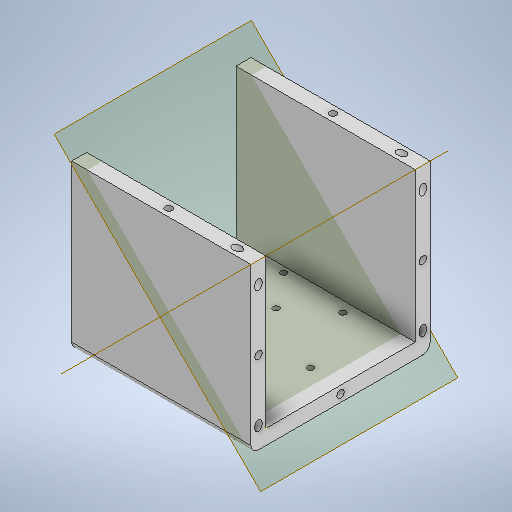
# Autodesk Inventor part: Fuselage_Body_Piece_Front
Saved by Autodesk Inventor 2025.1 (Build 291241020, 241B)
## iProperties
Created: 2025-02-15
Part Number: Fuselage_Body_Piece_Front
Material: Generic
Document SubType Name: Modeling
Designer: smyth
Density: 1 g/cm^3
Appearance: Default
Author: smyth
Autodesk Inventor part; units mm, degrees
ref_plane "YZ Plane" through (0, 0, 0) normal (1, 0, 0) x (0, 1, 0)
ref_plane "XZ Plane" through (0, 0, 0) normal (0, 1, 0) x (-1, 0, 0)
ref_plane "XY Plane" through (0, 0, 0) normal (0, 0, 1) x (1, 0, 0)
sketch "Sketch1" plane through (0, 0, 0) normal (0, 1, 0) x (-1, 0, 0)
  point P0 (0, 0)
sketch "Sketch2" plane through (0, 0, 0) normal (0, 1, 0) x (-1, 0, 0)
  line L0 (-76.2, 76.2) -> (76.2, 76.2)
  line L1 (76.2, 76.2) -> (76.2, -76.2)
  line L2 (76.2, -76.2) -> (-76.2, -76.2)
  line L3 (-76.2, -76.2) -> (-76.2, 76.2)
  line L4 (-76.2, 76.2) -> (76.2, -76.2) construction
  line L5 (76.2, 76.2) -> (-76.2, -76.2) construction
  point P0 (0, 0)
  dimension "d0" = 152.4
  dimension "d1" = 152.4
  constraints: 12 end point, 2 midpoint, 2 parallel, 1 horizontal, 1 perpendicular
  measures "d0" distance of L1.end L2.end
  measures "d1" distance of L0.end L1.end
extrude "Extrusion1" add sketch "Sketch2" along normal blind 12.7
sketch "Sketch3" plane through (0, 12.7, 0) normal (0, 1, 0) x (1, 0, 0)
  line L0 (76.2, 76.2) -> (-76.2, 76.2) projected
  line L1 (76.2, -76.2) -> (76.2, 76.2) projected
  line L2 (-76.2, 76.2) -> (76.2, 76.2)
  line L3 (76.2, 76.2) -> (76.2, 63.5)
  line L4 (76.2, 63.5) -> (-76.2, 63.5)
  line L5 (-76.2, 63.5) -> (-76.2, 76.2)
  line L6 (-76.2, -76.2) -> (76.2, -76.2)
  line L7 (76.2, -76.2) -> (76.2, -63.5)
  line L8 (76.2, -63.5) -> (-76.2, -63.5)
  line L9 (-76.2, -63.5) -> (-76.2, -76.2)
  point P0 (0, 0)
  point P1 (76.2, -76.2)
  dimension "d4" = 12.7
  dimension "d5" = 12.7
  dimension "d15" = 152.4
  constraints: 16 end point, 4 parallel, 2 horizontal, 2 perpendicular, 2 point on line
  measures "d4" distance between parallel lines of L4 L0
  measures "d5" distance between parallel lines of L8 L6
  measures "d15" distance of L6.start L6.end
extrude "Extrusion2" add sketch "Sketch3" along normal blind 127
fillet "Fillet1" radius 6.35 2 edges at (0, 0, 76.2) (0, 0, -76.2)
sketch "Sketch4" plane through (76.2, 12.7, -63.5) normal (1, 0, 0) x (0, 0, -1)
  circle A0 centre (-133.35, 57.15) radius 3.175
  circle A1 centre (6.35, 57.15) radius 3.175
  circle A2 centre (-63.5, -6.35) radius 3.175
  point P0 (-63.5, -12.7)
  constraints: 3 centre point
extrude "Extrusion3" cut sketch "Sketch4" against normal blind 12.7
sketch "Sketch5" plane through (-76.2, 12.7, 63.5) normal (-1, 0, 0) x (0, 0, 1)
  circle A0 centre (-133.35, 120.65) radius 3.175
  circle A1 centre (-133.35, 57.15) radius 3.175 projected
  circle A2 centre (-133.35, 57.15) radius 3.175
  circle A3 centre (-133.35, -6.35) radius 3.175
  circle A4 centre (-63.5, -6.35) radius 3.175 projected
  circle A5 centre (-63.5, -6.35) radius 3.175
  circle A6 centre (6.35, -6.35) radius 3.175
  circle A7 centre (6.35, 57.15) radius 3.175 projected
  circle A8 centre (6.35, 57.15) radius 3.175
  circle A9 centre (6.35, 120.65) radius 3.175
  line L0 (6.35, -12.7) -> (-133.35, -12.7) projected
  point P0 (-63.5, -12.7)
  point P1 (-133.35, 120.65)
  point P2 (-133.35, -6.35)
  point P3 (6.35, -6.35)
  point P4 (6.35, 120.65)
  dimension "d20" = 69.85
  constraints: 7 centre point, 7 coincident
  measures "d20" distance from line of L0 A8.centre
sketch "Sketch6" plane through (0, 139.7, 0) normal (0, 1, 0) x (1, 0, 0)
  line L0 (76.2, 69.85) -> (-76.2, 69.85) projected
  circle A0 centre (0, 69.85) radius 3
  line L1 (-76.2, -69.85) -> (76.2, -69.85) projected
  circle A1 centre (0, -69.85) radius 3
  point P0 (0, 0)
  dimension "d16" = 6
  dimension "d17" = 6
  constraints: 2 centre point, 2 midpoint
  measures "d16" diameter of A0
  measures "d17" diameter of A1
extrude "Extrusion5" cut sketch "Sketch6" against normal blind 4
extrude "Extrusion6" cut sketch "Sketch5" against normal blind 12.7 contours A1 | A4 | A7
ref_plane "Work Plane1" through (76.2, 139.7, 76.2) normal (0.7071, -0.7071, 0) x (0, 0, -1)
sketch "Sketch7" plane through (76.2, 139.7, 76.2) normal (0.7071, -0.7071, 0) x (0, 0, -1)
  line L0 (139.7, 0) -> (152.4, 0) projected
  line L1 (146.05, 0) -> (146.05, -12.7)
  circle A0 centre (146.05, -12.7) radius 3.175
  line L2 (0, 0) -> (12.7, 0) projected
  line L3 (6.35, 0) -> (6.35, -12.7)
  circle A1 centre (6.35, -12.7) radius 3.175
  point P0 (76.2, -152.6644)
  dimension "d24" = 12.7
  constraints: 4 end point, 2 centre point, 2 coincident, 2 midpoint, 2 vertical
  measures "d24" distance of L3.start L3.end
extrude "Extrusion7" cut sketch "Sketch7" along normal blind 31.75 and the other way blind 25.4
ref_plane "Work Plane2" through (76.2, 0, 76.2) normal (-0.7071, -0.7071, 0) x (0, 0, -1)
sketch "Sketch8" plane through (76.2, 0, 76.2) normal (-0.7071, -0.7071, 0) x (0, 0, -1)
  line L0 (6.35, 0) -> (146.05, 0) projected
  line L1 (146.05, 0) -> (146.05, -12.7)
  line L2 (146.05, 0) -> (146.05, -107.7631) projected
  line L3 (6.35, 0) -> (6.35, -12.7)
  line L4 (6.35, -107.7631) -> (6.35, 0) projected
  circle A0 centre (146.05, -12.7) radius 3.175
  circle A1 centre (6.35, -12.7) radius 3.175
  point P0 (76.2, -53.8815)
  dimension "d30" = 12.7
  dimension "d31" = 12.7
  constraints: 4 end point, 2 centre point, 2 coincident, 2 point on line
  measures "d30" distance of L0.end L1.end
  measures "d31" distance of L0.start L3.end
extrude "Extrusion8" cut sketch "Sketch8" along normal blind 25.4 and the other way blind 31.75
sketch "Sketch10" plane through (0, 12.7, 0) normal (0, 1, 0) x (1, 0, 0)
  line L0 (76.2, -63.5) -> (76.2, 63.5) projected
  line L1 (76.2, 0) -> (50.8, 0)
  circle A0 centre (50.8, 0) radius 2.6035
  line L2 (48.1965, 0) -> (-5.1435, 0)
  circle A1 centre (-7.747, 0) radius 2.6035
  line L3 (-5.1435, -17.8483) -> (-5.1435, 18.0947)
  line L4 (-5.1435, 0) -> (-5.1435, -49.2125)
  line L5 (23.8125, 0) -> (23.8125, -51.8414)
  line L6 (23.8125, 0) -> (23.8125, 51.8414)
  circle A2 centre (23.8125, -54.4449) radius 2.6035
  circle A3 centre (23.8125, 54.4449) radius 2.6035
  line L7 (30.1625, -51.8414) -> (15.875, -51.8414)
  line L8 (30.1625, 51.8414) -> (17.4625, 51.8414)
  point P0 (0, 0)
  dimension "d37" = 5.207
  dimension "d36" = 25.4
  dimension "d39" = 5.207
  dimension "d40" = 49.2125
  dimension "d41" = 51.8414
  dimension "d42" = 51.8414
  dimension "d43" = 5.207
  constraints: 16 end point, 4 horizontal, 3 centre point, 3 point on line, 3 tangent, 1 coincident, 1 horizontal alignment, 1 midpoint, 1 perpendicular, 1 vertical, 2 other
  measures "d36" distance of L1.start L1.end
  measures "d39" diameter of A1
  measures "d40" distance of L2.end L4.end
  measures "d41" distance of L5.start L5.end
  measures "d42" distance of L5.start L6.end
  measures "d43" diameter of A2
extrude "Extrusion9" cut sketch "Sketch10" against normal blind 3.9878
sketch "Sketch11" plane through (0, 12.7, 0) normal (0, 1, 0) x (1, 0, 0)
  circle A0 centre (-7.747, 0) radius 2.6035 projected
  line L0 (-10.3505, 29.2735) -> (-50.9905, 29.2735)
  line L1 (-63.5, -3.175) -> (-63.5, 3.175) projected
  line L2 (-50.8997, 16.5035) -> (-50.8997, 42.0435)
  circle A1 centre (-53.5032, 29.2735) radius 2.6035
  line L3 (-30.6705, 29.2735) -> (-30.6705, 2.6035)
  line L4 (-30.6705, 29.2735) -> (-30.6705, 55.9435)
  line L5 (-23.5267, 29.2578) -> (-40.9893, 29.2578)
  line L6 (-40.9893, 2.6035) -> (-17.4625, 2.6035)
  circle A2 centre (-30.6705, 0) radius 2.6035
  line L7 (-37.2049, 55.9435) -> (-23.5267, 55.9435)
  circle A3 centre (-30.6705, 58.547) radius 2.6035
  circle A4 centre (-7.747, 29.2578) radius 2.6035
  point P0 (0, 0)
  dimension "d46" = 40.64
  dimension "d47" = 5.207
  dimension "d48" = 26.67
  dimension "d49" = 26.67
  dimension "d59" = 5.207
  dimension "d60" = 5.207
  dimension "d61" = 5.207
  constraints: 14 end point, 4 centre point, 3 horizontal, 3 tangent, 3 vertical, 1 line through centre, 1 midpoint, 1 perpendicular
  measures "d46" distance of L0.start L0.end
  measures "d47" diameter of A1
  measures "d48" distance of L3.start L3.end
  measures "d49" distance of L3.start L4.end
  measures "d59" diameter of A2
  measures "d60" diameter of A3
  measures "d61" diameter of A4
extrude "Extrusion10" cut sketch "Sketch11" against normal blind 3.9878 contours A2 | A1 | A3 | A4
sketch "Sketch12" plane through (0, 12.7, 0) normal (0, 1, 0) x (1, 0, 0)
  point P0 (0, 0)
sketch "Sketch13" plane through (0, 12.7, 0) normal (0, 1, 0) x (1, 0, 0)
  circle A0 centre (-53.5032, 29.2735) radius 2.6035 projected
  circle A1 centre (-30.6705, 0) radius 2.6035 projected
  line L0 (-30.6705, -2.6035) -> (-30.6705, -38.1635)
  line L1 (-30.6705, -20.3835) -> (-43.3705, -20.3835)
  line L2 (-43.3705, -20.3835) -> (-17.9705, -20.3835)
  circle A2 centre (-45.974, -20.3835) radius 2.6035
  circle A3 centre (-15.367, -20.3835) radius 2.6035
  circle A4 centre (-30.6705, -40.767) radius 2.6035
  point P0 (0, 0)
  dimension "d65" = 5.207
  dimension "d66" = 5.207
  dimension "d67" = 5.207
  dimension "d62" = 35.56
  dimension "d63" = 12.7
  dimension "d64" = 25.4
  constraints: 6 end point, 2 horizontal alignment, 2 vertical alignment, 1 horizontal, 1 midpoint, 1 point on line, 1 vertical, 7 other
  measures "d62" distance of L0.start L0.end
  measures "d63" distance of L1.start L1.end
  measures "d64" distance of L1.end L2.end
extrude "Extrusion11" cut sketch "Sketch13" against normal blind 3.9878 contours A3 | A4 | A2
sketch "Sketch14" plane through (0, 12.7, 0) normal (0, 1, 0) x (1, 0, 0)
  line L0 (-76.2, -63.5) -> (76.2, -63.5) projected
  line L1 (-33.3375, -63.5) -> (-21.9075, -63.5)
  point P0 (0, 0)
  constraints: 2 end point, 2 point on line
body "Solid1"
